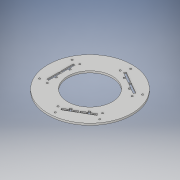
# Autodesk Inventor part: Stewart-Platform-Base-Außenanordnung
Saved by Autodesk Inventor 2018.2 (Build 222227000, 227)
## iProperties
Created: 2018-02-17
Part Number: Stewart-Platform-Base-Außenanordnung
Material: Generisch
Document SubType Name: Modeling
Designer: JochenAlt
Density: 1 g/cm^3
Appearance: Vorgabe
Author: JochenAlt
Autodesk Inventor part; units mm, degrees
ref_plane "YZ Plane" through (0, 0, 0) normal (1, 0, 0) x (0, 1, 0)
ref_plane "XZ Plane" through (0, 0, 0) normal (0, 1, 0) x (-1, 0, 0)
ref_plane "XY Plane" through (0, 0, 0) normal (0, 0, 1) x (1, 0, 0)
sketch "Skizze1" plane through (0, 0, 0) normal (0, 0, 1) x (1, 0, 0)
  line L0 (0, 95.3893) -> (0, -95.3893) construction
  line L1 (-95.3893, 0) -> (95.3893, 0) construction
  line L2 (-55.3629, 29.8) -> (-42.9629, 29.8) construction
  line L3 (-39.5629, 26.4) -> (-39.5629, -26.4) construction
  line L4 (-42.9629, -29.8) -> (-55.3629, -29.8) construction
  line L5 (-58.7629, -26.4) -> (-58.7629, 26.4) construction
  arc A0 (-55.3629, 29.8) -> (-58.7629, 26.4) centre (-55.3629, 26.4) ccw construction
  arc A1 (-39.5629, 26.4) -> (-42.9629, 29.8) centre (-42.9629, 26.4) ccw construction
  arc A2 (-42.9629, -29.8) -> (-39.5629, -26.4) centre (-42.9629, -26.4) ccw construction
  arc A3 (-58.7629, -26.4) -> (-55.3629, -29.8) centre (-55.3629, -26.4) ccw construction
  circle A4 centre (-55.3629, 26.4) radius 1.4
  circle A5 centre (-42.9629, 26.4) radius 1.4
  circle A6 centre (-55.3629, -26.4) radius 1.4
  circle A7 centre (-42.9629, -26.4) radius 1.4
  line L6 (-45.4629, 21.4) -> (-45.4629, -21.4)
  line L7 (-48.7629, 21.4) -> (-48.7629, -21.4)
  line L8 (-48.7629, 21.4) -> (-45.4629, 21.4)
  line L9 (-48.7629, -21.4) -> (-45.4629, -21.4)
  line L10 (-48.7629, 0.8) -> (-45.4629, 0.8)
  line L11 (-48.7629, -0.8) -> (-45.4629, -0.8)
  line L12 (-45.4629, 12.5) -> (-42.5469, 12.5)
  line L13 (-42.5469, 12.5) -> (-42.5469, 9.7)
  line L14 (-42.5469, 9.7) -> (-45.4629, 9.7)
  line L15 (-45.4629, -9.7) -> (-42.5469, -9.7)
  line L16 (-42.5469, -9.7) -> (-42.5469, -12.5)
  line L17 (-42.5469, -12.5) -> (-45.4629, -12.5)
  line L18 (-42.9629, 30.2) -> (-55.3629, 30.2)
  arc A8 (-55.3629, 30.2) -> (-59.1629, 26.4) centre (-55.3629, 26.4) ccw
  line L19 (-59.1629, 26.4) -> (-59.1629, -26.4)
  arc A9 (-59.1629, -26.4) -> (-55.3629, -30.2) centre (-55.3629, -26.4) ccw
  line L20 (-55.3629, -30.2) -> (-42.9629, -30.2)
  arc A10 (-42.9629, -30.2) -> (-39.1629, -26.4) centre (-42.9629, -26.4) ccw
  line L21 (-39.1629, -26.4) -> (-39.1629, 26.4)
  arc A11 (-39.1629, 26.4) -> (-42.9629, 30.2) centre (-42.9629, 26.4) ccw
  line L22 (-61.2675, -29.7727) -> (-58.6625, -28.2847) construction
  line L23 (42.9144, -31.5299) -> (41.2644, -28.672)
  circle A12 centre (44.3445, -24.0069) radius 1.4
  arc A13 (47.289, -22.3069) -> (42.6445, -21.0624) centre (44.3445, -24.0069) ccw construction
  arc A14 (47.6354, -22.1069) -> (42.4445, -20.716) centre (44.3445, -24.0069) ccw
  circle A15 centre (50.5445, -34.7456) radius 1.4
  line L24 (56.4177, -38.1729) -> (53.8266, -36.6608) construction
  arc A16 (52.2445, -37.6901) -> (53.489, -33.0456) centre (50.5445, -34.7456) ccw construction
  arc A17 (52.4445, -38.0365) -> (53.8354, -32.8456) centre (50.5445, -34.7456) ccw
  line L25 (53.8354, -32.8456) -> (47.6354, -22.1069)
  line L26 (47.289, -22.3069) -> (53.489, -33.0456) construction
  line L27 (1.8739, -62.8456) -> (-4.3261, -52.1069) construction
  arc A18 (1.8739, -62.8456) -> (6.5184, -64.0901) centre (4.8184, -61.1456) ccw construction
  circle A19 centre (4.8184, -61.1456) radius 1.4
  circle A20 centre (-1.3816, -50.4069) radius 1.4
  arc A21 (1.5275, -63.0456) -> (6.7184, -64.4365) centre (4.8184, -61.1456) ccw
  line L28 (-4.6725, -52.3069) -> (1.5275, -63.0456)
  arc A22 (-3.0816, -47.4624) -> (-4.3261, -52.1069) centre (-1.3816, -50.4069) ccw construction
  arc A23 (-3.2816, -47.116) -> (-4.6725, -52.3069) centre (-1.3816, -50.4069) ccw
  line L29 (32.0987, -30.5967) -> (33.5567, -33.122)
  line L30 (29.6739, -31.9967) -> (32.0987, -30.5967)
  line L31 (31.1319, -34.522) -> (29.6739, -31.9967)
  line L32 (5.8485, -52.9299) -> (4.1985, -50.072)
  line L33 (11.9061, -45.622) -> (10.4481, -43.0967)
  line L34 (10.4481, -43.0967) -> (12.873, -41.6967)
  line L35 (12.873, -41.6967) -> (14.331, -44.222)
  line L36 (23.6886, -42.6299) -> (22.0386, -39.772)
  line L37 (25.0742, -41.8299) -> (23.4242, -38.972)
  line L38 (4.1985, -50.072) -> (41.2644, -28.672)
  line L39 (42.4445, -20.716) -> (-3.2816, -47.116)
  line L40 (-3.0816, -47.4624) -> (42.6445, -21.0624) construction
  line L41 (52.2445, -37.6901) -> (6.5184, -64.0901) construction
  line L42 (6.7184, -64.4365) -> (52.4445, -38.0365)
  line L43 (5.8485, -52.9299) -> (42.9144, -31.5299)
  line L44 (5.8485, 52.9299) -> (4.1985, 50.072)
  circle A24 centre (-1.3816, 50.4069) radius 1.4
  arc A25 (-4.3261, 52.1069) -> (-3.0816, 47.4624) centre (-1.3816, 50.4069) ccw construction
  arc A26 (-4.6725, 52.3069) -> (-3.2816, 47.116) centre (-1.3816, 50.4069) ccw
  circle A27 centre (4.8184, 61.1456) radius 1.4
  line L45 (4.8498, 67.9456) -> (4.8359, 64.9456) construction
  arc A28 (6.5184, 64.0901) -> (1.8739, 62.8456) centre (4.8184, 61.1456) ccw construction
  arc A29 (6.7184, 64.4365) -> (1.5275, 63.0456) centre (4.8184, 61.1456) ccw
  line L46 (1.5275, 63.0456) -> (-4.6725, 52.3069)
  line L47 (-4.3261, 52.1069) -> (1.8739, 62.8456) construction
  line L48 (53.489, 33.0456) -> (47.289, 22.3069) construction
  arc A30 (53.489, 33.0456) -> (52.2445, 37.6901) centre (50.5445, 34.7456) ccw construction
  circle A31 centre (50.5445, 34.7456) radius 1.4
  circle A32 centre (44.3445, 24.0069) radius 1.4
  arc A33 (53.8354, 32.8456) -> (52.4445, 38.0365) centre (50.5445, 34.7456) ccw
  line L49 (47.6354, 22.1069) -> (53.8354, 32.8456)
  arc A34 (42.6445, 21.0624) -> (47.289, 22.3069) centre (44.3445, 24.0069) ccw construction
  arc A35 (42.4445, 20.716) -> (47.6354, 22.1069) centre (44.3445, 24.0069) ccw
  line L50 (10.4481, 43.0967) -> (11.9061, 45.622)
  line L51 (12.873, 41.6967) -> (10.4481, 43.0967)
  line L52 (14.331, 44.222) -> (12.873, 41.6967)
  line L53 (42.9144, 31.5299) -> (41.2644, 28.672)
  line L54 (33.5567, 33.122) -> (32.0987, 30.5967)
  line L55 (32.0987, 30.5967) -> (29.6739, 31.9967)
  line L56 (29.6739, 31.9967) -> (31.1319, 34.522)
  line L57 (25.0742, 41.8299) -> (23.4242, 38.972)
  line L58 (23.6886, 42.6299) -> (22.0386, 39.772)
  line L59 (41.2644, 28.672) -> (4.1985, 50.072)
  line L60 (-3.2816, 47.116) -> (42.4445, 20.716)
  line L61 (42.6445, 21.0624) -> (-3.0816, 47.4624) construction
  line L62 (6.5184, 64.0901) -> (52.2445, 37.6901) construction
  line L63 (52.4445, 38.0365) -> (6.7184, 64.4365)
  line L64 (42.9144, 31.5299) -> (5.8485, 52.9299)
  line L65 (-36.1629, 0) -> (-39.1629, 0) construction
  circle A36 centre (0, 0) radius 36.1629
  circle A37 centre (0, 0) radius 68.1352
  line L66 (-61.5007, 29.3269) -> (-58.7928, 28.0356) construction
  line L67 (-42.5469, -11.1) -> (-6.4086, -11.1) construction
  line L68 (11.6605, -42.3967) -> (-6.4086, -11.1) construction
  line L69 (-38.1629, -11.1) -> (-38.1629, -66.1) construction
  line L70 (9.4685, -38.6) -> (-38.1629, -66.1) construction
  dimension "d43" = 136.2704
  dimension "d1" = 59.6
  dimension "d2" = 19.2
  dimension "d3" = 3.4
  dimension "d5" = 2.8
  dimension "d6" = 5.9
  dimension "d7" = 3.3
  dimension "d8" = 20.6
  dimension "d9" = 1.6
  dimension "d10" = 2.984
  dimension "d11" = 2.8
  dimension "d12" = 19.4
  dimension "d21" = 0.4
  dimension "d22" = 3
  dimension "d32" = 360
  dimension "d34" = 3
  dimension "d35" = 3
  dimension "d40" = 1
  dimension "d41" = 1
  dimension "d42" = 55
  constraints: 138 end point, 52 point on circle, 36 centre point, 27 point on line, 14 coincident, 9 perpendicular, 8 tangent, 7 horizontal, 6 equal radius, 4 midpoint, 4 parallel, 3 vertical, 2 line through centre, 1 collinear, 1 horizontal alignment, 244 other
  measures "d1" distance between parallel lines of L4 L2
  measures "d2" distance between parallel lines of L3 L5
  measures "d3" radius of A0
  measures "d5" diameter of A4
  measures "d6" distance between parallel lines of L3 L6
  measures "d7" distance between parallel lines of L6 L7
  measures "d8" distance between parallel lines of L10 L8
  measures "d9" distance between parallel lines of L11 L10
  measures "d10" distance between parallel lines of L3 L13
  measures "d11" distance between parallel lines of L14 L12
  measures "d12" distance between parallel lines of L15 L14
  measures "d21" distance between parallel lines of L19 L5
  measures "d22" distance of L22.end L22.start
  measures "d34" distance of L65.start L65.end
  measures "d35" distance of L66.start L66.end
  measures "d40" distance between parallel lines of L21 L69
  measures "d41" distance between parallel lines of L70 L39
  measures "d42" distance from line of L67 L69.end
extrude "Extrusion5" add sketch "Skizze1" along normal blind 3 contours L10 L6 L11 L7 | A11 L21 A10 L20 A9 L19 A8 L18 | L43 L36 L38 L37 | L25 A17 L42 A21 L28 A23 L39 A14 | L64 L57 L59 L58 | L46 A29 L63 A33 L49 A35 L60 A26 | A37
extrude "Extrusion4" cut sketch "Skizze1" along normal blind 1 contours L10 L6 L11 L7 | A11 L21 A10 L20 A9 L19 A8 L18 | L43 L36 L38 L37 | L25 A17 L42 A21 L28 A23 L39 A14 | L64 L57 L59 L58 | L46 A29 L63 A33 L49 A35 L60 A26
equation "\"d22\" = d20"
equation "\"d35\" = d34"
equation "\"d41\" = d40"
equation "\"d20\" = 3"
